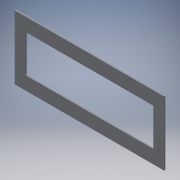
# Autodesk Inventor part: LFEV2017_TSI_003
Saved by Autodesk Inventor 2017 (Build 210142000, 142)
## iProperties
Created: 2017-04-03
Part Number: LFEV2017_TSI_003
Material: Generic
Document SubType Name: Modeling
Designer: hoeflinc
Density: 1 g/cm^3
Appearance: Default
Material_size: Steel   Thickness: .125"
Quantity: 1
Author: hoeflinc
Autodesk Inventor part; units mm, degrees
ref_plane "YZ Plane" through (0, 0, 0) normal (1, 0, 0) x (0, 1, 0)
ref_plane "XZ Plane" through (0, 0, 0) normal (0, 1, 0) x (-1, 0, 0)
ref_plane "XY Plane" through (0, 0, 0) normal (0, 0, 1) x (1, 0, 0)
sketch "Sketch1" plane through (0, 0, 0) normal (0, 0, 1) x (1, 0, 0)
  line L0 (0, 0) -> (355.6, 0)
  line L1 (355.6, 0) -> (355.6, 152.4)
  line L2 (355.6, 152.4) -> (0, 152.4)
  line L3 (0, 152.4) -> (0, 0)
  dimension "d0" = 152.4
  dimension "d1" = 355.6
  constraints: 8 end point, 2 parallel, 1 horizontal, 1 perpendicular
  measures "d0" distance of L2.end L0.start
  measures "d1" distance of L0.start L0.end
extrude "Extrusion1" add sketch "Sketch1" along normal blind 3.175
sketch "Sketch2" plane through (0, 0, 3.175) normal (0, 0, 1) x (1, 0, 0)
  line L0 (355.6, 0) -> (355.6, 152.4) projected
  line L1 (0, 152.4) -> (0, 0) projected
  line L2 (355.6, 152.4) -> (0, 152.4) projected
  line L3 (0, 0) -> (355.6, 0) projected
  point P0 (12.7, 31.75)
  point P1 (12.7, 120.65)
  point P2 (342.9, 120.65)
  point P3 (342.9, 31.75)
  dimension "d4" = 12.7
  dimension "d5" = 12.7
  dimension "d6" = 12.7
  dimension "d7" = 12.7
  dimension "d8" = 31.75
  dimension "d9" = 31.75
  dimension "d10" = 31.75
  dimension "d11" = 31.75
  measures "d4" distance from line of point (342.9, 120.65) L0
  measures "d5" distance from line of point (342.9, 31.75) L0
  measures "d6" distance from line of point (12.7, 31.75) L1
  measures "d7" distance from line of point (12.7, 120.65) L1
  measures "d8" distance from line of point (342.9, 120.65) L2
  measures "d9" distance from line of point (12.7, 120.65) L2
  measures "d10" distance from line of point (342.9, 31.75) L3
  measures "d11" distance from line of point (12.7, 31.75) L3
hole "Hole1" at (12.7, 31.75, 3.175) at (12.7, 120.65, 3.175) at (342.9, 120.65, 3.175) at (342.9, 31.75, 3.175) direction (0, 0, -1) diameter 3.302 end through all thread size "8-32 UNC" class "2B" standard "ANSI Unified Screw Threads"
sketch "Sketch3" plane through (0, 0, 3.175) normal (0, 0, 1) x (1, 0, 0)
  line L0 (25.4, 31.75) -> (330.2, 31.75)
  line L1 (330.2, 31.75) -> (330.2, 120.65)
  line L2 (330.2, 120.65) -> (25.4, 120.65)
  line L3 (25.4, 120.65) -> (25.4, 31.75)
  line L4 (0, 152.4) -> (0, 0) projected
  circle A0 centre (342.9, 120.65) radius 1.651 projected
  circle A1 centre (12.7, 31.75) radius 1.651 projected
  circle A2 centre (12.7, 120.65) radius 1.651 projected
  circle A3 centre (342.9, 31.75) radius 1.651 projected
  line L5 (0, 0) -> (355.6, 0) projected
  line L6 (355.6, 0) -> (355.6, 152.4) projected
  line L7 (355.6, 152.4) -> (0, 152.4) projected
  line L8 (0, 152.4) -> (0, 0) projected
  dimension "d27" = 25.4
  dimension "d28" = 304.8
  dimension "d29" = 31.75
  dimension "d30" = 88.9
  constraints: 8 end point, 2 parallel, 1 horizontal, 1 perpendicular
  measures "d27" distance between parallel lines of L4 L3
  measures "d28" distance of L0.start L0.end
  measures "d29" distance between parallel lines of L0 L5
  measures "d30" distance of L0.end L1.end
extrude "Extrusion2" cut sketch "Sketch3" against normal blind 3.175 contours L3 L2 L1 L0
fillet "Fillet1" radius 3.175 4 edges at (25.4, 31.75, 1.5875) (25.4, 120.65, 1.5875) (330.2, 120.65, 1.5875) (330.2, 31.75, 1.5875)
equation "\"d5\" = d4"
equation "\"d6\" = d4"
equation "\"d7\" = d4"
equation "\"d9\" = d8"
equation "\"d10\" = d8"
equation "\"d11\" = d8"
body "Solid1"
